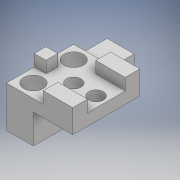
# Autodesk Inventor part: SensorMount
Saved by Autodesk Inventor 2018 (Build 220112000, 112)
## iProperties
Created: 2018-05-09
Part Number: SensorMount
Material: Generic
Document SubType Name: Modeling
Designer: s4321966
Mass: 0.48957 g
Surface Area: 8.77183 cm^2
Volume: 0.48957 cm^3
Density: 1 g/cm^3
Appearance: Default
Author: s4321966
Autodesk Inventor part; units mm, degrees
ref_plane "YZ Plane" through (0, 0, 0) normal (1, 0, 0) x (0, 1, 0)
ref_plane "XZ Plane" through (0, 0, 0) normal (0, 1, 0) x (-1, 0, 0)
ref_plane "XY Plane" through (0, 0, 0) normal (0, 0, 1) x (1, 0, 0)
sketch "Sketch21" plane through (0, 0, 0) normal (0, 0, 1) x (1, 0, 0)
  line L0 (0, 0) -> (0, 6.858)
  line L1 (0, 6.858) -> (3.429, 6.858)
  line L2 (3.429, 6.858) -> (3.429, 3.434)
  line L3 (3.429, 3.434) -> (7.229, 3.434)
  circle A0 centre (0, 0) radius 1.651
  circle A1 centre (0, 6.858) radius 1.651
  circle A2 centre (3.429, 3.434) radius 1.25
  circle A3 centre (7.229, 3.434) radius 1.25
  line L4 (7.229, 3.434) -> (8.979, 3.434)
  line L5 (8.979, 9.144) -> (-2.286, 9.144)
  line L6 (-2.286, 9.144) -> (-2.286, -2.286)
  line L7 (-2.286, -2.286) -> (8.979, -2.286)
  line L8 (8.979, -2.286) -> (8.979, 9.144)
  dimension "d76" = 6.858
  dimension "d77" = 3.429
  dimension "d78" = 3.424
  dimension "d79" = 3.8
  dimension "d80" = 3.302
  dimension "d81" = 3.302
  dimension "d82" = 2.5
  dimension "d83" = 2.5
  dimension "d84" = 1.75
  constraints: 18 end point, 4 centre point, 4 coincident, 3 horizontal, 3 perpendicular, 2 parallel, 1 vertical
  measures "d76" distance of L0.start L0.end
  measures "d77" distance of L0.end L1.end
  measures "d78" distance of L1.end L2.end
  measures "d79" distance of L2.end L3.end
  measures "d80" diameter of A0
  measures "d81" diameter of A1
  measures "d82" diameter of A2
  measures "d83" diameter of A3
  measures "d84" distance of L4.start L4.end
extrude "Extrusion19" add sketch "Sketch21" along normal blind 2
sketch "Sketch22" plane through (0, 0, 2) normal (0, 0, 1) x (1, 0, 0)
  line L0 (-2.286, -2.286) -> (8.979, -2.286) projected
  line L1 (8.979, -2.286) -> (3.979, -2.286)
  line L2 (3.979, -2.286) -> (3.979, 0.214)
  line L3 (3.979, 0.214) -> (8.979, 0.214)
  line L4 (8.979, 0.214) -> (8.979, -2.286)
  line L5 (8.979, 9.144) -> (-2.286, 9.144) projected
  line L6 (8.979, 9.144) -> (3.979, 9.144)
  line L7 (3.979, 9.144) -> (3.979, 6.644)
  line L8 (3.979, 6.644) -> (8.979, 6.644)
  line L9 (8.979, 6.644) -> (8.979, 9.144)
  line L10 (-2.286, 9.144) -> (-2.286, -2.286) projected
  line L11 (-2.286, 3.429) -> (-1.286, 3.429)
  line L12 (-1.286, 3.429) -> (-1.286, 4.429)
  line L13 (-1.286, 4.429) -> (-2.286, 4.429)
  line L14 (-2.286, 4.429) -> (-2.286, 3.429)
  line L15 (-2.286, 4.429) -> (-0.286, 4.429)
  line L16 (-0.286, 4.429) -> (-0.286, 2.429)
  line L17 (-0.286, 2.429) -> (-2.286, 2.429)
  line L18 (-2.286, 2.429) -> (-2.286, 4.429)
  point P0 (0, 0)
  dimension "d89" = 5
  dimension "d90" = 2.5
  dimension "d91" = 5
  dimension "d92" = 2.5
  dimension "d93" = 1
  dimension "d94" = 1
  dimension "d95" = 2
  dimension "d96" = 2
  constraints: 32 end point, 8 parallel, 4 horizontal, 4 perpendicular, 1 midpoint
  measures "d89" distance of L2.end L3.end
  measures "d90" distance of L1.end L2.end
  measures "d91" distance of L8.end L7.end
  measures "d92" distance of L7.end L6.end
  measures "d93" distance of L13.end L12.end
  measures "d94" distance of L12.end L11.end
  measures "d95" distance of L16.end L17.end
  measures "d96" distance of L15.end L16.end
extrude "Extrusion20" add sketch "Sketch22" along normal blind 2
sketch "Sketch23" plane through (0, 0, 0) normal (0, 0, -1) x (-1, 0, 0)
  circle A0 centre (0, 6.858) radius 1.651 projected
  circle A1 centre (0, 6.858) radius 2.286
  line L0 (2.286, 9.144) -> (2.286, -2.286) projected
  line L1 (-2.286, 6.858) -> (-2.286, -2.286)
  line L2 (-8.979, 9.144) -> (2.286, 9.144) projected
  line L3 (-2.286, -2.286) -> (2.286, -2.286)
  line L4 (2.286, -2.286) -> (2.286, 9.144)
  line L5 (2.286, 9.144) -> (-2.286, 9.144)
  line L6 (-2.286, 9.144) -> (-2.286, -2.286)
  circle A2 centre (0, 0) radius 1.651
  constraints: 10 end point, 3 vertical, 2 coincident, 2 parallel, 1 centre point, 1 horizontal, 1 horizontal alignment, 1 perpendicular, 2 other
extrude "Extrusion21" add sketch "Sketch23" along normal blind 5
sketch "Sketch24" plane through (2.286, 2.928, 0) normal (1, 0, 0) x (0, 0, -1)
  line L0 (5, -5.214) -> (5, 6.216) projected
  line L1 (5, 6.216) -> (-2, 6.216) projected
  line L2 (5, -5.214) -> (5, 6.216)
  line L3 (5, 0.501) -> (-9.7149, 0.501)
  line L4 (0, 1.012) -> (0, 0) projected
  line L5 (0, 0.506) -> (5, 0.501)
  circle A0 centre (2.5, 0.5035) radius 1.651
  point P0 (0, -2.928)
  dimension "d101" = 3.302
  constraints: 6 end point, 3 midpoint, 1 centre point, 1 horizontal, 1 perpendicular
  measures "d101" diameter of A0
extrude "Extrusion22" cut sketch "Sketch24" against normal blind 5 contours A0 L3 | L3 A0
sketch "Sketch25" plane through (2.286, 2.928, 0) normal (1, 0, 0) x (0, 0, -1)
  circle A0 centre (2.5, 0.5035) radius 1.651 projected
  line L0 (5, 6.216) -> (-2, 6.216) projected
  line L1 (5, -5.214) -> (5, 6.216) projected
  circle A1 centre (2.5, 9.0723) radius 1.651
  line L2 (5, 11.9285) -> (0, 11.9285)
  line L3 (0, 11.9285) -> (0, 6.216)
  line L4 (0, 6.216) -> (5, 6.216)
  line L5 (5, 6.216) -> (5, 11.9285)
  point P0 (0, -2.928)
  dimension "d105" = 3.302
  constraints: 8 end point, 2 parallel, 1 centre point, 1 horizontal, 1 perpendicular
  measures "d105" diameter of A1
extrude "Extrusion23" add sketch "Sketch25" against normal blind 5 contours L0 L3 L2 L5
sketch "Sketch26" plane through (-2.714, 9.144, 0) normal (0, -1, 0) x (1, 0, 0)
  line L0 (0.428, 0) -> (0, 0) projected
  line L1 (5, -5) -> (0.428, -5) projected
  line L2 (0, 0) -> (0.428, 0)
  line L3 (0.428, 0) -> (0.428, -5)
  line L4 (0.428, -5) -> (0, -5)
  line L5 (0, -5) -> (0, 0)
  point P0 (2.714, 0)
  constraints: 8 end point, 2 parallel, 1 horizontal, 1 perpendicular
extrude "Extrusion24" cut sketch "Sketch26" against normal blind 50
body "Solid2"
